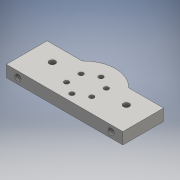
# Autodesk Inventor part: motormt
Saved by Autodesk Inventor 2016 (Build 200138000, 138)
## iProperties
Created: 2016-09-01
Part Number: motormt
Material: 一般
Document SubType Name: Modeling
Designer: KOTA-NPC2
Density: 1 g/cm^3
Appearance: 既定
Author: KOTA-NPC2
Autodesk Inventor part; units mm, degrees
ref_plane "YZ Plane" through (0, 0, 0) normal (1, 0, 0) x (0, 1, 0)
ref_plane "XZ Plane" through (0, 0, 0) normal (0, 1, 0) x (-1, 0, 0)
ref_plane "XY Plane" through (0, 0, 0) normal (0, 0, 1) x (1, 0, 0)
sketch "構築線" plane through (0, 0, 0) normal (0, 0, 1) x (1, 0, 0)
  circle A0 centre (0, 0) radius 2.75 construction
  circle A1 centre (0, 0) radius 8.5 construction
  line L0 (-33.6576, -8.5) -> (34.6793, -8.5) construction
  line L1 (-34.7345, -10) -> (33.6024, -10) construction
  line L2 (-34.854, 1) -> (33.4828, 1) construction
  line L3 (-33.6339, 12) -> (34.7029, 12) construction
  circle A2 centre (12.7107, 1) radius 10 construction
  circle A3 centre (-12.7107, 1) radius 10 construction
  circle A4 centre (12.7107, 1) radius 11 construction
  circle A5 centre (-12.7107, 1) radius 11 construction
  circle A6 centre (0, 0) radius 5 construction
  line L4 (0, 0) -> (0, 6) construction
  circle A7 centre (0, 5) radius 0.8
  line L5 (0, 0) -> (-5.1962, 3) construction
  circle A8 centre (-4.3301, 2.5) radius 0.8
  circle A9 centre (0, 0) radius 5 construction
  line L6 (0, 0) -> (-5.1962, -3) construction
  circle A10 centre (-4.3301, -2.5) radius 0.8
  circle A11 centre (0, 0) radius 5 construction
  line L7 (0, 0) -> (0, -6) construction
  circle A12 centre (0, -5) radius 0.8
  circle A13 centre (0, 0) radius 5 construction
  line L8 (0, 0) -> (5.1962, -3) construction
  circle A14 centre (4.3301, -2.5) radius 0.8
  circle A15 centre (0, 0) radius 5 construction
  line L9 (0, 0) -> (5.1962, 3) construction
  circle A16 centre (4.3301, 2.5) radius 0.8
  circle A17 centre (0, 0) radius 5 construction
  circle A18 centre (-12.7107, 1) radius 1.05
  circle A19 centre (12.7107, 1) radius 1.05
  line L10 (-20, 6.5) -> (-8, 6.5)
  line L11 (20, 6.5) -> (8, 6.5)
  arc A20 (8, 6.5) -> (-8, 6.5) centre (0, -1.0498) ccw
  line L12 (-33.6339, -7.5) -> (34.7029, -7.5) construction
  line L13 (-20, 6.5) -> (-20, -7.5)
  line L14 (20, 6.5) -> (20, -7.5)
  line L15 (-20, -7.5) -> (20, -7.5)
  dimension "d51" = 10
  dimension "d0" = 5.5
  dimension "d1" = 17
  dimension "d12" = 20
  dimension "d13" = 20
  dimension "d14" = 11
  dimension "d15" = 8.5
  dimension "d16" = 11
  dimension "d17" = 1.5
  dimension "d18" = 22
  dimension "d19" = 22
  dimension "d54" = 1.6
  dimension "d57" = 360
  dimension "d59" = 2.1
  dimension "d61" = 2.1
  dimension "d65" = 12
  dimension "d66" = 12
  dimension "d70" = 11
  dimension "d71" = 1
  dimension "d72" = 14
  dimension "d73" = 14
  dimension "d75" = 20
  dimension "d76" = 20
  constraints: 32 end point, 15 centre point, 11 point on line, 7 coincident, 6 horizontal, 2 concentric, 2 perpendicular, 2 point on circle, 2 tangent, 2 vertical alignment, 1 collinear, 1 vertical, 51 other
  measures "d0" diameter of A0
  measures "d1" diameter of A1
  measures "d12" diameter of A2
  measures "d13" diameter of A3
  measures "d14" distance between parallel lines of L1 L2
  measures "d15" distance from line of point (0, 0) L0
  measures "d16" distance between parallel lines of L2 L3
  measures "d17" distance between parallel lines of L1 L0
  measures "d18" diameter of A4
  measures "d19" diameter of A5
  measures "d54" diameter of A7
  measures "d59" diameter of A18
  measures "d61" diameter of A19
  measures "d65" distance of L10.start L10.end
  measures "d66" distance of L11.start L11.end
  measures "d70" radius of A20
  measures "d71" distance between parallel lines of L0 L12
  measures "d72" distance between parallel lines of L10 L12
  measures "d73" distance between parallel lines of L12 L11
  measures "d75" distance from line of point (0, 0) L13
  measures "d76" distance from line of point (0, 0) L14
extrude "押し出し1" add sketch "構築線" along normal mid plane 4
sketch "スケッチ5" plane through (-20, -7.5, 2) normal (0, -1, 0) x (1, 0, 0)
  circle A0 centre (4, -2) radius 1.05
  circle A1 centre (36, -2) radius 1.05
  line L0 (0, 0) -> (40, 0) projected
  point P0 (20, -2)
  dimension "d88" = 2.1
  dimension "d89" = 2.1
  dimension "d90" = 16
  dimension "d92" = 2
  dimension "d93" = 16
  dimension "d94" = 2
  constraints: 2 centre point
  measures "d88" diameter of A1
  measures "d89" diameter of A0
  measures "d90" distance of point (20, -2) A1.centre
  measures "d92" distance from line of A1.centre L0
  measures "d93" distance of point (20, -2) A0.centre
  measures "d94" distance from line of L0 A0.centre
extrude "押し出し3" cut sketch "スケッチ5" against normal blind 4
thread "ねじ3" size "M2.2x0.45" class "6H" standard "ANSI Metric M Profile" full length
thread "ねじ4" size "M2.2x0.45" class "6H" standard "ANSI Metric M Profile" full length
